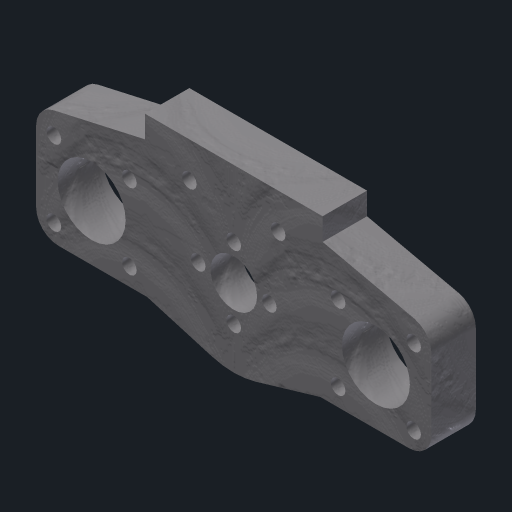
# Autodesk Inventor part: PARA_TUERCA
Saved by Autodesk Inventor 2024.3 (Build 283343000, 343)
## iProperties
Created: 2024-08-24
Part Number: PARA_TUERCA
Material: Steel, Mild, Welded
Document SubType Name: Modeling
Designer: Niler
Density: 7.85 g/cm^3
Appearance: Weld - Steel Mild
Author: Niler
Autodesk Inventor part; units mm, degrees
ref_plane "YZ Plane" through (0, 0, 0) normal (1, 0, 0) x (0, 1, 0)
ref_plane "XZ Plane" through (0, 0, 0) normal (0, 1, 0) x (-1, 0, 0)
ref_plane "XY Plane" through (0, 0, 0) normal (0, 0, 1) x (1, 0, 0)
sketch "Sketch1" plane through (0, 0, 0) normal (0, 0, 1) x (1, 0, 0)
  line L0 (-20, -5) -> (20, -5)
  line L1 (20, -5) -> (20, 5)
  line L2 (20, 5) -> (-20, 5)
  line L3 (-20, 5) -> (-20, -5)
  line L4 (-20, -5) -> (20, 5) construction
  line L5 (20, -5) -> (-20, 5) construction
  circle A0 centre (0, -18) radius 11.15
  circle A1 centre (0, -18) radius 5.25
  circle A2 centre (0, -18) radius 17.5
  line L6 (-20, -5) -> (-17.2455, -20.9738)
  line L7 (20, -5) -> (17.2455, -20.9738)
  circle A3 centre (0, -10) radius 1.65
  circle A4 centre (-8, -18) radius 1.65
  circle A5 centre (0, -26) radius 1.65
  circle A6 centre (8, -18) radius 1.65
  circle A7 centre (32, -18) radius 7.65
  line L8 (19.5, -30.5) -> (44.5, -30.5)
  line L9 (44.5, -30.5) -> (44.5, -5.5)
  line L10 (44.5, -5.5) -> (19.5, -5.5)
  line L11 (19.5, -5.5) -> (19.5, -30.5)
  line L12 (19.5, -30.5) -> (44.5, -5.5) construction
  line L13 (44.5, -30.5) -> (19.5, -5.5) construction
  circle A8 centre (23.5, -9.5) radius 1.65
  circle A9 centre (40.5, -9.5) radius 1.65
  circle A10 centre (40.5, -26.5) radius 1.65
  circle A11 centre (23.5, -26.5) radius 1.65
  line L14 (44.5, -5.5) -> (20, 0)
  line L15 (19.5, -30.5) -> (4.9442, -34.787)
  line L16 (0, 5) -> (0, 15.3431)
  circle A12 centre (-32, -18) radius 7.65
  line L17 (-19.5, -30.5) -> (-44.5, -30.5)
  line L18 (-44.5, -30.5) -> (-44.5, -5.5)
  line L19 (-44.5, -5.5) -> (-19.5, -5.5)
  line L20 (-19.5, -5.5) -> (-19.5, -30.5)
  line L21 (-19.5, -30.5) -> (-44.5, -5.5) construction
  line L22 (-44.5, -30.5) -> (-19.5, -5.5) construction
  circle A13 centre (-23.5, -9.5) radius 1.65
  circle A14 centre (-40.5, -9.5) radius 1.65
  circle A15 centre (-40.5, -26.5) radius 1.65
  circle A16 centre (-23.5, -26.5) radius 1.65
  line L23 (-44.5, -5.5) -> (-20, 0)
  line L24 (-19.5, -30.5) -> (-4.9442, -34.787)
  point P0 (0, 0)
  point P1 (-4.9442, -34.787)
  dimension "d0" = 22.3
  dimension "d1" = 10.5
  dimension "d2" = 35
  dimension "d3" = 3.3
  dimension "d4" = 8
  dimension "d7" = 360
  dimension "d14" = 40
  dimension "d16" = 23
  dimension "d17" = 10
  dimension "d24" = 15.3
  dimension "d25" = 32
  dimension "d27" = 25
  dimension "d28" = 25
  dimension "d29" = 3.3
  dimension "d30" = 17
  constraints: 50 end point, 17 centre point, 11 symmetric about line, 8 point on line, 6 midpoint, 4 parallel, 4 vertical alignment, 3 equal radius, 3 horizontal alignment, 3 point on circle, 3 tangent, 2 coincident, 2 horizontal, 2 perpendicular, 1 vertical, 14 other
  measures "d0" diameter of A0
  measures "d1" diameter of A1
  measures "d2" diameter of A2
  measures "d3" diameter of A3
  measures "d4" distance of A0.centre A3.centre
  measures "d14" distance of L1.end L2.end
  measures "d16" distance from line of A0.centre L2
  measures "d17" distance of L2.end L0.start
  measures "d24" diameter of A7
  measures "d25" distance of A7.centre A1.centre
  measures "d27" distance of L10.end L9.end
  measures "d28" distance of L9.end L8.end
  measures "d29" diameter of A8
  measures "d30" distance of A9.centre A8.centre
extrude "Extrusion1" add sketch "Sketch1" along normal blind 10 contours L3 L2 L1 L0 A2 | L0 A2 L6 L20 L19 | A2 L0 | L0 A2 | L19 L20 L6 | L0 L7 L10 L11 A2 | L7 L11 L10 | A0
extrude "Extrusion2" cut sketch "Sketch1" along normal blind 3 contours A0
sketch "Sketch2" plane through (0, 0, 10) normal (0, 0, 1) x (1, 0, 0)
  line L0 (20, 5) -> (-20, 5) projected
  line L1 (-20, 5) -> (-20, -5) projected
  line L2 (-20, -5) -> (-17.2455, -20.9738) projected
  arc A0 (-17.2455, -20.9738) -> (17.2455, -20.9738) centre (0, -18) ccw projected
  line L3 (17.2455, -20.9738) -> (20, -5) projected
  line L4 (20, -5) -> (20, 5) projected
  circle A1 centre (0, -18) radius 5.25 projected
  circle A2 centre (0, -10) radius 1.65 projected
  circle A3 centre (-8, -18) radius 1.65 projected
  circle A4 centre (0, -26) radius 1.65 projected
  circle A5 centre (8, -18) radius 1.65 projected
  circle A6 centre (-10, -3) radius 1.65
  circle A7 centre (10, -3) radius 1.65
  line L5 (-10, -3) -> (10, -3)
  point P0 (0, 0)
  point P1 (0, -3)
  dimension "d18" = 3.3
  dimension "d19" = 3.3
  dimension "d20" = 8
  dimension "d21" = 20
  constraints: 2 centre point, 2 end point, 1 horizontal, 1 horizontal alignment, 1 midpoint, 1 vertical alignment
  measures "d18" diameter of A6
  measures "d19" diameter of A7
  measures "d20" distance between parallel lines of L0 L5
  measures "d21" distance of L5.start L5.end
extrude "Extrusion3" cut sketch "Sketch2" against normal through all contours A6 | A7
extrude "Extrusion4" add sketch "Sketch1" along normal blind 10 contours L6 L19 L23 L3 | L6 L20 L17 L18 L19 | A2 L24 L20 L6 | L1 L14 L10 L7 | L10 L9 L8 L11 L7 | L7 L11 L15 A2
fillet "Fillet1" radius 5 4 edges at (-44.5, -5.5, 5) (-44.5, -30.5, 5) (44.5, -30.5, 5) (44.5, -5.5, 5)
body "Solid1"
